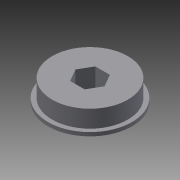
# Autodesk Inventor part: Bearing
Saved by Autodesk Inventor 2013 (Build 170138000, 138)
## iProperties
Created: 2013-01-16
Part Number: Bearing
Material: Generic
Document SubType Name: Modeling
Designer: actoennies
Density: 1 g/cm^3
Mass: 4.21214 g
Surface Area: 23.7987 cm^2
Volume: 4.21214 cm^3
Author: actoennies
Autodesk Inventor part; units mm, degrees
ref_plane "YZ Plane" through (0, 0, 0) normal (1, 0, 0) x (0, 1, 0)
ref_plane "XZ Plane" through (0, 0, 0) normal (0, 1, 0) x (-1, 0, 0)
ref_plane "XY Plane" through (0, 0, 0) normal (0, 0, 1) x (1, 0, 0)
sketch "Sketch1" plane through (0, 0, 0) normal (0, 1, 0) x (-1, 0, 0)
  circle A0 centre (0, 0) radius 15.875
  line L0 (2.7496, 4.7625) -> (5.4993, 0)
  line L1 (5.4993, 0) -> (2.7496, -4.7625)
  line L2 (2.7496, -4.7625) -> (-2.7496, -4.7625)
  line L3 (-2.7496, -4.7625) -> (-5.4993, 0)
  line L4 (-5.4993, 0) -> (-2.7496, 4.7625)
  line L5 (-2.7496, 4.7625) -> (2.7496, 4.7625)
  dimension "d0" = 31.75
  dimension "d9" = 9.525
  constraints: 12 end point, 2 coincident, 1 centre point, 13 other
  measures "d0" diameter of A0
  measures "d9" distance between parallel lines of L2 L5
extrude "Extrusion1" add sketch "Sketch1" along normal blind 1.397
sketch "Sketch2" plane through (0, 1.397, 0) normal (0, 1, 0) x (1, 0, 0)
  line L0 (-5.4993, 0) -> (-2.7496, 4.7625) projected
  line L1 (-2.7496, 4.7625) -> (2.7496, 4.7625) projected
  line L2 (2.7496, 4.7625) -> (5.4993, 0) projected
  line L3 (5.4993, 0) -> (2.7496, -4.7625) projected
  line L4 (2.7496, -4.7625) -> (-2.7496, -4.7625) projected
  line L5 (-2.7496, -4.7625) -> (-5.4993, 0) projected
  circle A0 centre (0, 0) radius 15.875 projected
  circle A1 centre (0, 0) radius 14.2875
  dimension "d6" = 28.575
  constraints: 1 centre point, 1 coincident
  measures "d6" diameter of A1
extrude "Extrusion2" add sketch "Sketch2" along normal blind 6.5278 contours A1
body "Solid1"
